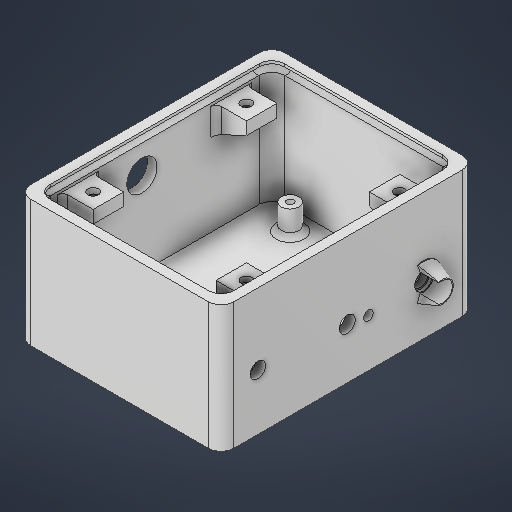
# Autodesk Inventor part: Box
Saved by Autodesk Inventor 2026 (Build 300175000, 175)
## iProperties
Created: 2025-05-11
Part Number: Box
Material: ABS Plastic
Document SubType Name: Modeling
Designer: Riley
Density: 1.06 g/cm^3
Appearance: Smooth - White
Author: Riley
Autodesk Inventor part; units mm, degrees
sketch "Sketch1" plane through (0, 0, 0) normal (0, 1, 0) x (-1, 0, 0)
  line L0 (0, 0) -> (100, 0)
  line L1 (100, 0) -> (100, -80)
  line L2 (100, -80) -> (0, -80)
  line L3 (0, -80) -> (0, 0)
  dimension "d0" = 100
  dimension "d1" = 80
  constraints: 8 end point, 2 parallel, 1 horizontal, 1 perpendicular
  measures "d0" distance of L1.end L2.end
  measures "d1" distance of L0.end L1.end
extrude "BoxProfile" add sketch "Sketch1" along normal blind 50
sketch "Sketch2" plane through (0, 0, 0) normal (0, -1, 0) x (1, 0, 0)
  line L0 (-3.8, -3.8) -> (-96.2, -3.8)
  line L1 (-96.2, -3.8) -> (-96.2, -76.2)
  line L2 (-96.2, -76.2) -> (-3.8, -76.2)
  line L3 (-3.8, -76.2) -> (-3.8, -3.8)
  line L4 (0, -80) -> (-100, -80) projected
  line L5 (0, 0) -> (0, -80) projected
  line L6 (-100, 0) -> (0, 0) projected
  line L7 (-100, -80) -> (-100, 0) projected
  dimension "d4" = 3.8
  dimension "d5" = 3.8
  dimension "d6" = 3.8
  dimension "d7" = 3.8
  constraints: 8 end point, 2 parallel, 1 horizontal, 1 perpendicular
  measures "d4" distance between parallel lines of L5 L3
  measures "d5" distance between parallel lines of L6 L0
  measures "d6" distance between parallel lines of L4 L2
  measures "d7" distance between parallel lines of L7 L1
extrude "Walls" cut sketch "Sketch2" against normal blind 48 contours L3 L2 L1 L0
fillet "Fillet1" radius 5 8 edges at (0, 25, 0) (0, 25, -80) (-100, 25, 0) (-100, 25, -80) (-96.2, 24, -76.2) (-96.2, 24, -3.8) (-3.8, 24, -3.8) (-3.8, 24, -76.2)
ref_plane "Work Plane1" through (0, 5, 0) normal (0, -1, 0) x (1, 0, 0)
sketch "Sketch3" plane through (0, 5, 0) normal (0, -1, 0) x (1, 0, 0)
  arc A0 (-8.8, -76.2) -> (-3.8, -71.2) centre (-8.8, -71.2) ccw projected
  line L0 (-3.8, -8.8) -> (-3.8, -71.2) projected
  arc A1 (-3.8, -8.8) -> (-8.8, -3.8) centre (-8.8, -8.8) ccw projected
  line L1 (-91.2, -3.8) -> (-8.8, -3.8) projected
  arc A2 (-91.2, -3.8) -> (-96.2, -8.8) centre (-91.2, -8.8) ccw projected
  line L2 (-96.2, -71.2) -> (-96.2, -8.8) projected
  arc A3 (-96.2, -71.2) -> (-91.2, -76.2) centre (-91.2, -71.2) ccw projected
  line L3 (-8.8, -76.2) -> (-91.2, -76.2) projected
  line L4 (-13.8, -3.8) -> (-25.8, -3.8)
  line L5 (-25.8, -3.8) -> (-25.8, -15.8)
  line L6 (-25.8, -15.8) -> (-13.8, -15.8)
  line L7 (-13.8, -15.8) -> (-13.8, -3.8)
  line L8 (2.9782, -40) -> (-105.6038, -40) construction
  line L9 (-95, 0) -> (-5, 0) projected
  line L10 (-50, 11.1583) -> (-50, -101.8999) construction
  line L11 (0, -5) -> (0, -75) projected
  line L12 (-13.8, -3.8) -> (-25.8, -3.8)
  line L13 (-102.9782, -40) -> (5.6038, -40) construction
  line L14 (-13.8, -76.2) -> (-25.8, -76.2)
  line L15 (-86.2, -76.2) -> (-78.2, -76.2)
  circle A4 centre (-19.8, -9.8) radius 2.1
  point P0 (0, 0)
  point P1 (-25.8, -3.8)
  dimension "d12" = 12
  dimension "d13" = 12
  dimension "d14" = 40
  dimension "d15" = 50
  dimension "d16" = 10
  dimension "d19" = 6
  dimension "d20" = 6
  dimension "d21" = 4.2
  constraints: 20 end point, 4 symmetric about line, 2 horizontal, 2 parallel, 1 centre point, 1 coincident, 1 collinear, 1 perpendicular, 1 point on line, 1 vertical
  measures "d12" distance of L6.end L5.end
  measures "d13" distance of L5.end L4.end
  measures "d14" distance between parallel lines of L9 L8
  measures "d15" distance between parallel lines of L11 L10
  measures "d16" distance between parallel lines of L0 L7
  measures "d19" distance from line of L7 point (-19.8, -9.8)
  measures "d20" distance from line of L6 point (-19.8, -9.8)
  measures "d21" diameter of A4
extrude "ScrewPosts" add sketch "Sketch3" against normal blind 5 contours L7 L6 L5 L1
sketch "Sketch5" plane through (-25.8, 5, -15.8) normal (-1, 0, 0) x (0, 0, 1)
  line L0 (-60.4, 43) -> (-60.4, -5) projected
  line L1 (-60.4, -5) -> (-64.2, -5) projected
  line L2 (-64.2, -5) -> (-64.2, 45) projected
  line L3 (-64.2, 45) -> (15.8, 45) projected
  line L4 (15.8, 45) -> (15.8, -5) projected
  line L5 (15.8, -5) -> (12, -5) projected
  line L6 (12, -5) -> (12, 0) projected
  line L7 (12, 0) -> (0, 0) projected
  line L8 (0, 0) -> (0, 5) projected
  line L9 (0, 5) -> (12, 5) projected
  line L10 (12, 5) -> (12, 43) projected
  line L11 (12, 43) -> (-60.4, 43) projected
  line L12 (12, 5) -> (12, 0) projected
  line L13 (12, 5) -> (0, 5) projected
  line L14 (0, 5) -> (12, 10.5957)
  line L15 (12, 5) -> (12, 10.5957)
  line L16 (0, 5) -> (12, 5)
  point P0 (15.8, -5)
  dimension "d23" = 25
  constraints: 6 end point, 1 collinear, 1 point on line
  measures "d23" angle of L9 L14
extrude "PrintSlope" add sketch "Sketch5" against normal up to surface (12 mm away) contours L10 L9 L14
ref_plane "Work Plane2" through (-25.8, 10, -15.8) normal (0, -1, 0) x (-1, 0, 0)
sketch "Sketch6" plane through (-25.8, 10, -15.8) normal (0, -1, 0) x (-1, 0, 0)
  circle A0 centre (-6, -6) radius 2.1 projected
  arc A1 (-22, -7) -> (-17, -12) centre (-17, -7) ccw projected
  line L0 (-17, -12) -> (-12, -12) projected
  line L1 (-12, -12) -> (-12, 0) projected
  line L2 (-12, 0) -> (0, 0) projected
  line L3 (0, 0) -> (0, -12) projected
  line L4 (0, -12) -> (65.4, -12) projected
  arc A2 (65.4, -12) -> (70.4, -7) centre (65.4, -7) ccw projected
  line L5 (70.4, -7) -> (70.4, 55.4) projected
  arc A3 (70.4, 55.4) -> (65.4, 60.4) centre (65.4, 55.4) ccw projected
  line L6 (65.4, 60.4) -> (-17, 60.4) projected
  arc A4 (-17, 60.4) -> (-22, 55.4) centre (-17, 55.4) ccw projected
  line L7 (-22, 55.4) -> (-22, -7) projected
  arc A5 (-20.8, 64.2) -> (-25.8, 59.2) centre (-20.8, 59.2) ccw projected
  line L8 (-20.8, 64.2) -> (69.2, 64.2) projected
  arc A6 (74.2, 59.2) -> (69.2, 64.2) centre (69.2, 59.2) ccw projected
  line L9 (74.2, 59.2) -> (74.2, -10.8) projected
  arc A7 (69.2, -15.8) -> (74.2, -10.8) centre (69.2, -10.8) ccw projected
  line L10 (69.2, -15.8) -> (-20.8, -15.8) projected
  arc A8 (-25.8, -10.8) -> (-20.8, -15.8) centre (-20.8, -10.8) ccw projected
  line L11 (-25.8, -10.8) -> (-25.8, 59.2) projected
  line L12 (-3.8638, -9.7) -> (-8.1362, -9.7)
  line L13 (-8.1362, -9.7) -> (-10.2724, -6)
  line L14 (-10.2724, -6) -> (-8.1362, -2.3)
  line L15 (-8.1362, -2.3) -> (-3.8638, -2.3)
  line L16 (-3.8638, -2.3) -> (-1.7276, -6)
  line L17 (-1.7276, -6) -> (-3.8638, -9.7)
  point P0 (-25.8, -15.8)
  dimension "d27" = 7.4
  dimension "d29" = 7.4
  dimension "d30" = 7.4
  dimension "d32" = 3.7
  dimension "d33" = 3.7
  constraints: 12 end point, 3 equal length, 3 parallel, 1 coincident, 1 horizontal
  measures "d27" distance between parallel lines of L15 L12
  measures "d29" distance between parallel lines of L13 L16
  measures "d30" distance between parallel lines of L17 L14
  measures "d32" distance from line of L15 point (-6, -6)
  measures "d33" distance from line of L17 point (-6, -6)
extrude "HexNut" cut sketch "Sketch6" along normal blind 2.8 contours L12 L13 L14 L15 L16 L17
sketch "Sketch7" plane through (-25.8, 10, -15.8) normal (0, -1, 0) x (-1, 0, 0)
  line L0 (-3.8638, -9.7) -> (-1.7276, -6) projected
  line L1 (-1.7276, -6) -> (-3.8638, -2.3) projected
  line L2 (-3.8638, -2.3) -> (-8.1362, -2.3) projected
  line L3 (-8.1362, -2.3) -> (-10.2724, -6) projected
  line L4 (-10.2724, -6) -> (-8.1362, -9.7) projected
  line L5 (-8.1362, -9.7) -> (-3.8638, -9.7) projected
  arc A0 (-22, -7) -> (-17, -12) centre (-17, -7) ccw projected
  line L6 (-17, -12) -> (-12, -12) projected
  line L7 (-12, -12) -> (-12, 0) projected
  line L8 (-12, 0) -> (0, 0) projected
  line L9 (0, 0) -> (0, -12) projected
  line L10 (0, -12) -> (65.4, -12) projected
  arc A1 (65.4, -12) -> (70.4, -7) centre (65.4, -7) ccw projected
  line L11 (70.4, -7) -> (70.4, 55.4) projected
  arc A2 (70.4, 55.4) -> (65.4, 60.4) centre (65.4, 55.4) ccw projected
  line L12 (65.4, 60.4) -> (-17, 60.4) projected
  arc A3 (-17, 60.4) -> (-22, 55.4) centre (-17, 55.4) ccw projected
  line L13 (-22, 55.4) -> (-22, -7) projected
  arc A4 (-20.8, 64.2) -> (-25.8, 59.2) centre (-20.8, 59.2) ccw projected
  line L14 (-20.8, 64.2) -> (69.2, 64.2) projected
  arc A5 (74.2, 59.2) -> (69.2, 64.2) centre (69.2, 59.2) ccw projected
  line L15 (74.2, 59.2) -> (74.2, -10.8) projected
  arc A6 (69.2, -15.8) -> (74.2, -10.8) centre (69.2, -10.8) ccw projected
  line L16 (69.2, -15.8) -> (-20.8, -15.8) projected
  arc A7 (-25.8, -10.8) -> (-20.8, -15.8) centre (-20.8, -10.8) ccw projected
  line L17 (-25.8, -10.8) -> (-25.8, 59.2) projected
  line L18 (65.4, -12) -> (-17, -12) projected
  line L19 (-0.8, -12) -> (-11.2, -12)
  line L20 (-11.2, -12) -> (-11.2, 0)
  line L21 (-11.2, 0) -> (-0.8, 0)
  line L22 (-0.8, 0) -> (-0.8, -12)
  point P0 (-25.8, -15.8)
  point P1 (-0.8, 0)
  dimension "d36" = 0.8
  dimension "d37" = 0.8
  constraints: 8 end point, 2 parallel, 2 point on line, 1 horizontal, 1 perpendicular
  measures "d36" distance between parallel lines of L9 L22
  measures "d37" distance between parallel lines of L7 L20
extrude "SupportCut" cut sketch "Sketch7" against normal blind 10 contours L5 L4 L3 L2 L1 L0 | L20 L8 L22 L18
pattern_linear "Rectangular Pattern1" count 2 spacing -60.4 along (1, 0, 0) of "ScrewPosts", "PrintSlope", "HexNut", "SupportCut"
fillet "Fillet3" radius 2 4 edges at (-25.8, 10.2978, -3.8) (-13.8, 10.2978, -3.8) (-86.2, 10.2978, -3.8) (-74.2, 10.2978, -3.8)
ref_plane "Work Plane3" through (-5, 0, -40) normal (0, 0, -1) x (-1, 0, 0)
sketch "Sketch8" plane through (-5, 0, -40) normal (0, 0, -1) x (-1, 0, 0)
  line L0 (-1.2, 0) -> (-5, 0) projected
  line L1 (-5, 0) -> (-5, 50) projected
  line L2 (-5, 50) -> (95, 50) projected
  line L3 (95, 50) -> (95, 0) projected
  line L4 (95, 0) -> (91.2, 0) projected
  line L5 (91.2, 0) -> (91.2, 48) projected
  line L6 (91.2, 48) -> (-1.2, 48) projected
  line L7 (-1.2, 48) -> (-1.2, 0) projected
  circle A0 centre (92.1, 2.5) radius 1.7
  dimension "d44" = 3.4
  dimension "d45" = 2.5
  dimension "d46" = 0.9
  constraints: 1 centre point
  measures "d44" diameter of A0
  measures "d45" distance from line of L4 A0.centre
  measures "d46" distance from line of L5 A0.centre
mirror "Mirror2" about plane through (-5, 0, -40) normal (0, 0, -1) of "ScrewPosts", "PrintSlope", "HexNut", "SupportCut", "Rectangular Pattern1", "Fillet3"
sketch3d "3D Sketch2"
  line L0 (-96.2, 0, -8.8) -> (-96.2, 0, -71.2)
  arc A0 (-96.2, 0, -71.2) -> (-91.2, 0, -76.2) centre (-91.2, 0, -71.2) ccw
  line L1 (-91.2, 0, -76.2) -> (-8.8, 0, -76.2)
  arc A1 (-8.8, 0, -76.2) -> (-3.8, 0, -71.2) centre (-8.8, 0, -71.2) ccw
  line L2 (-3.8, 0, -71.2) -> (-3.8, 0, -8.8)
  arc A2 (-3.8, 0, -8.8) -> (-8.8, 0, -3.8) centre (-8.8, 0, -8.8) ccw
  line L3 (-8.8, 0, -3.8) -> (-91.2, 0, -3.8)
  arc A3 (-91.2, 0, -3.8) -> (-96.2, 0, -8.8) centre (-91.2, 0, -8.8) ccw
sweep "oring groove" cut profiles "Sketch8" path "3D Sketch2" contours A0 L5 | L5 A0
sketch "Sketch9" plane through (0, 48, 0) normal (0, -1, 0) x (1, 0, 0)
  line L0 (-91.2, -76.2) -> (-8.8, -76.2) projected
  arc A0 (-8.8, -76.2) -> (-3.8, -71.2) centre (-8.8, -71.2) ccw projected
  line L1 (-3.8, -71.2) -> (-3.8, -8.8) projected
  arc A1 (-3.8, -8.8) -> (-8.8, -3.8) centre (-8.8, -8.8) ccw projected
  line L2 (-8.8, -3.8) -> (-91.2, -3.8) projected
  arc A2 (-91.2, -3.8) -> (-96.2, -8.8) centre (-91.2, -8.8) ccw projected
  line L3 (-96.2, -8.8) -> (-96.2, -71.2) projected
  arc A3 (-96.2, -71.2) -> (-91.2, -76.2) centre (-91.2, -71.2) ccw projected
  arc A4 (-5, -80) -> (0, -75) centre (-5, -75) ccw projected
  line L4 (-5, -80) -> (-95, -80) projected
  arc A5 (-100, -75) -> (-95, -80) centre (-95, -75) ccw projected
  line L5 (-100, -75) -> (-100, -5) projected
  arc A6 (-95, 0) -> (-100, -5) centre (-95, -5) ccw projected
  line L6 (-95, 0) -> (-5, 0) projected
  arc A7 (0, -5) -> (-5, 0) centre (-5, -5) ccw projected
  line L7 (0, -5) -> (0, -75) projected
  circle A8 centre (-11.8, -69.2) radius 3.5
  circle A9 centre (-11.8, -19) radius 3.5
  circle A10 centre (-77, -69.2) radius 3.5
  circle A11 centre (-77, -19) radius 3.5
  point P0 (0, 0)
  dimension "d52" = 7
  dimension "d53" = 7
  dimension "d54" = 7
  dimension "d55" = 7
  dimension "d56" = 8
  dimension "d57" = 7
  dimension "d58" = 65.2
  dimension "d59" = 50.2
  constraints: 4 centre point, 2 horizontal alignment, 2 vertical alignment
  measures "d52" diameter of A8
  measures "d53" diameter of A9
  measures "d54" diameter of A11
  measures "d55" diameter of A10
  measures "d56" distance from line of L1 A8.centre
  measures "d57" distance from line of L0 A8.centre
  measures "d58" distance of A8.centre A10.centre
  measures "d59" distance of A9.centre A8.centre
extrude "PCB posts" add sketch "Sketch9" along normal blind 10 contours A8 | A9 | A10 | A11
sketch "Sketch10" plane through (-11.8, 38, -19) normal (0, -1, 0) x (1, 0, 0)
  circle A0 centre (0, 0) radius 3.5 projected
  circle A1 centre (0, -50.2) radius 3.5 projected
  circle A2 centre (-65.2, 0) radius 3.5 projected
  circle A3 centre (0, -50.2) radius 3.5 projected
  circle A4 centre (-65.2, -50.2) radius 3.5 projected
  circle A5 centre (0, 0) radius 3.5 projected
  line L0 (-79.4, -57.2) -> (3, -57.2) projected
  arc A6 (3, -57.2) -> (8, -52.2) centre (3, -52.2) ccw projected
  line L1 (8, -52.2) -> (8, 10.2) projected
  arc A7 (8, 10.2) -> (3, 15.2) centre (3, 10.2) ccw projected
  line L2 (3, 15.2) -> (-79.4, 15.2) projected
  arc A8 (-79.4, 15.2) -> (-84.4, 10.2) centre (-79.4, 10.2) ccw projected
  line L3 (-84.4, 10.2) -> (-84.4, -52.2) projected
  arc A9 (-84.4, -52.2) -> (-79.4, -57.2) centre (-79.4, -52.2) ccw projected
  arc A10 (6.8, -61) -> (11.8, -56) centre (6.8, -56) ccw projected
  line L4 (6.8, -61) -> (-83.2, -61) projected
  arc A11 (-88.2, -56) -> (-83.2, -61) centre (-83.2, -56) ccw projected
  line L5 (-88.2, -56) -> (-88.2, 14) projected
  arc A12 (-83.2, 19) -> (-88.2, 14) centre (-83.2, 14) ccw projected
  line L6 (-83.2, 19) -> (6.8, 19) projected
  arc A13 (11.8, 14) -> (6.8, 19) centre (6.8, 14) ccw projected
  line L7 (11.8, 14) -> (11.8, -56) projected
  point P0 (11.8, 19)
  point P1 (-65.2, -50.2)
  constraints: 4 coincident
hole "Hole1" at (-11.8, 38, -19) at (-11.8, 38, -69.2) at (-77, 38, -69.2) at (-77, 38, -19) direction (0, 1, 0) diameter 2.8 depth 10.4
fillet "Fillet4" radius 2 4 edges at (-15.3, 48, -19) (-15.3, 48, -69.2) (-80.5, 48, -19) (-80.5, 48, -69.2)
sketch "Sketch11" plane through (-5, 0, -80) normal (0, 0, -1) x (-1, 0, 0)
  line L0 (68.5, 38) -> (75.5, 38) projected
  line L1 (3.3, 38) -> (10.3, 38) projected
  line L2 (-1.2, 48) -> (-1.2, 3.9422) projected
  line L3 (-1.2, 3.9422) -> (-1.2, 48) projected
  line L4 (91.2, 48) -> (91.2, 3.9422) projected
  line L5 (91.2, 3.9422) -> (91.2, 48) projected
  circle A0 centre (15.3, 30.2) radius 2.9
  line L6 (8.2, 38) -> (5.4, 38) projected
  line L7 (8.2, 38) -> (5.4, 38) projected
  line L8 (5.4, 48.4) -> (8.2, 48.4) projected
  line L9 (73.4, 38) -> (70.6, 38) projected
  line L10 (70.6, 48.4) -> (73.4, 48.4) projected
  circle A1 centre (37, 31.2) radius 1.9
  circle A2 centre (45.3, 30) radius 3.15
  circle A3 centre (80.5, 28) radius 3
  line L11 (8.2, 38) -> (5.4, 38) projected
  line L12 (3.3, 38) -> (10.3, 38) projected
  point P0 (-5, 0)
  point P1 (6.8, 38)
  point P2 (6.8, 38)
  point P3 (6.8, 38)
  point P4 (72, 38)
  point P5 (72, 38)
  dimension "d70" = 8.5
  dimension "d71" = 5.8
  dimension "d72" = 7.8
  dimension "d73" = 3.8
  dimension "d74" = 6.3
  dimension "d75" = 30.2
  dimension "d76" = 38.5
  dimension "d78" = 10
  dimension "d79" = 6
  dimension "d123" = 8
  dimension "d124" = 6.8
  dimension "d126" = 5
  constraints: 5 midpoint, 4 centre point
  measures "d70" horizontal distance of point (6.8, 38) A0.centre
  measures "d71" diameter of A0
  measures "d72" distance from line of L1 A0.centre
  measures "d73" diameter of A1
  measures "d74" diameter of A2
  measures "d75" horizontal distance of A1.centre point (6.8, 38)
  measures "d76" horizontal distance of A2.centre point (6.8, 38)
  measures "d78" vertical distance of point (72, 38) A3.centre
  measures "d79" diameter of A3
  measures "d123" distance from line of L1 A2.centre
  measures "d124" distance from line of L1 A1.centre
  measures "d126" horizontal distance of L0.end A3.centre
extrude "Laser holes" cut sketch "Sketch11" against normal blind 6.3
sketch "Sketch12" plane through (-95, 0, 0) normal (0, 0, 1) x (1, 0, 0)
  line L0 (0, 0) -> (0, 50) projected
  line L1 (0, 0) -> (90, 0) projected
  line L2 (90, 50) -> (90, 0) projected
  line L3 (0, 50) -> (90, 50) projected
  circle A0 centre (40, 15) radius 6
  point P0 (95, 0)
  dimension "d82" = 12
  dimension "d83" = 50
  dimension "d98" = 35
  constraints: 1 centre point
  measures "d82" diameter of A0
  measures "d83" distance from line of L2 A0.centre
  measures "d98" distance from line of L3 A0.centre
extrude "connector" cut sketch "Sketch12" against normal blind 6.3 contours A0
ref_plane "Work Plane4" through (0, 8, 0) normal (0, -1, 0) x (1, 0, 0)
ref_plane "Work Plane5" through (0, 25, 0) normal (0, -1, 0) x (1, 0, 0)
sketch "Sketch14" plane through (-5, 0, -80) normal (0, 0, -1) x (-1, 0, 0)
  circle A0 centre (15.3, 30.2) radius 2.9 projected
  arc A1 (16.6339, 33.8648) -> (16.6339, 26.5352) centre (15.3, 30.2) ccw
  arc A2 (17.6599, 36.6839) -> (17.6599, 23.7161) centre (15.3, 30.2) ccw
  line L0 (15.3, 30.2) -> (6.5373, 30.2) construction
  line L1 (16.6339, 33.8648) -> (17.6599, 36.6839)
  line L2 (16.6339, 26.5352) -> (17.6599, 23.7161)
  line L3 (15.3, 30.2) -> (16.6339, 26.5352) construction
  point P0 (-5, 0)
  dimension "d112" = 1
  dimension "d113" = 3
  dimension "d133" = 110
  dimension "d134" = 110
  dimension "d135" = 110
  constraints: 8 end point, 4 point on circle, 2 centre point, 1 horizontal, 1 vertical alignment
  measures "d112" radial gap between concentric circles of A0 A1
  measures "d113" radial gap between concentric circles of A1 A2
  measures "d133" angle of L3 L0
  measures "d134" angle of L0 L2
  measures "d135" angle of L0 L1
extrude "Hood" add sketch "Sketch14" along normal blind 7.5 contours A1 L2 A2 L1
chamfer "Chamfer3" distance 7.2 angle 20 1 edges at (-13.4, 30.2, -87.5) measured on face at (-22.1343, 36.8517, -82.5)
sketch "Sketch16" plane through (-5, 0, -80) normal (0, 0, -1) x (-1, 0, 0)
  circle A0 centre (15.3, 30.2) radius 2.9 projected
  circle A1 centre (15.3, 30.2) radius 3.5
  point P0 (-5, 0)
  dimension "d130" = 7
  constraints: 1 centre point, 1 coincident
  measures "d130" diameter of A1
extrude "FilterHole" cut sketch "Sketch16" against normal blind 1.2 contours A0 | A1
sketch "Sketch17" plane through (-91.2, 48, -76.2) normal (0, 0, 1) x (1, 0, 0)
  line L0 (75.9, -10) -> (82.9, -10) projected
  line L1 (15.6, -10) -> (12.8, -10) projected
  line L2 (10.7, -10) -> (17.7, -10) projected
  line L3 (60.9609, -12.4) -> (59.3609, -12.4)
  line L4 (59.3609, -12.4) -> (59.3609, -24.4)
  line L5 (59.3609, -24.4) -> (60.9609, -24.4)
  line L6 (60.9609, -24.4) -> (60.9609, -12.4)
  point P0 (91.2, -48)
  point P1 (60.1609, -12.4)
  dimension "d136" = 1.6
  dimension "d137" = 12
  dimension "d138" = 2.4
  constraints: 8 end point, 2 parallel, 1 horizontal, 1 midpoint, 1 perpendicular
  measures "d136" distance of L5.end L4.end
  measures "d137" distance of L4.end L3.end
  measures "d138" distance from line of point (60.161, -12.4) L0
extrude "InteriorBlocker" add sketch "Sketch17" along normal blind 6
chamfer "Chamfer4" distance 6 angle 30 1 edges at (-31.0391, 35.6, -70.2) measured on face at (-30.7725, 35.6, -74.2)
equation "\"d5\" = d4"
equation "\"d6\" = d4"
equation "\"d7\" = d4"
equation "\"d13\" = d12"
equation "\"d14\" = 0.5 * d1"
equation "\"d15\" = 0.5 * d0"
equation "\"d19\" = 0.5 * d12"
equation "\"d20\" = d19"
equation "\"d29\" = d27"
equation "\"d30\" = d29"
equation "\"d32\" = 0.5 * d27"
equation "\"d33\" = d32"
equation "\"d37\" = d36"
equation "\"d53\" = d52"
equation "\"d54\" = d52"
equation "\"d55\" = d52"
equation "\"d80\" = d74"
equation "\"d84\" = d74"
body "Solid1"
